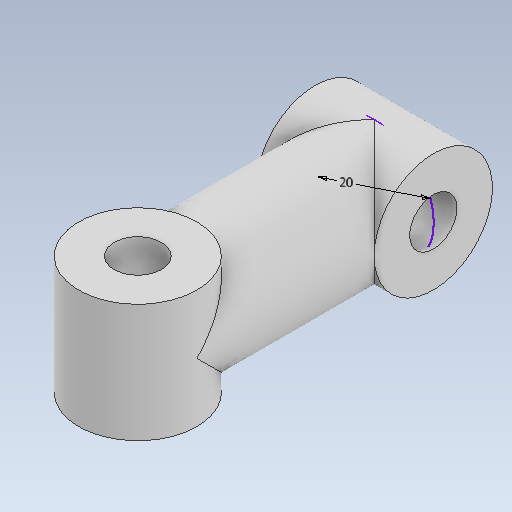
# Autodesk Inventor part: 10-06-007
Saved by Autodesk Inventor 2020 (Build 240168000, 168)
## iProperties
Created: 2019-11-09
Part Number: 10-06-007
Material: Generic
Document SubType Name: Modeling
Designer: iuliu
Density: 1 g/cm^3
Appearance: Default
Description: Suport display
Mass: 17.7888 g
Surface Area: 54.8743 cm^2
Volume: 17.7888 cm^3
Author: iuliu
Subject: 044
Autodesk Inventor part; units mm, degrees
ref_plane "YZ Plane" through (0, 0, 0) normal (1, 0, 0) x (0, 1, 0)
ref_plane "Work Plane2" through (0, 0, 10) normal (0, 0, 1) x (1, 0, 0)
sketch "Sketch2" plane through (0, 0, 10) normal (0, 0, 1) x (1, 0, 0)
  circle A0 centre (0, 0) radius 10
  dimension "d7" = 20
  constraints: 1 centre point
  measures "d7" diameter of A0
extrude "Extrusion2" add sketch "Sketch2" along normal blind 40
ref_plane "Work Plane1" through (0, -10, 0) normal (0, 1, 0) x (-1, 0, 0)
sketch "Sketch4" plane through (0, -10, 0) normal (0, 1, 0) x (-1, 0, 0)
  circle A0 centre (0, 50) radius 10
  line L0 (0, 10) -> (0, 50) projected
  line L1 (0, 10) -> (0, 50) projected
  circle A1 centre (0, 10) radius 10
  point P0 (0, 0)
  dimension "d12" = 20
  constraints: 2 centre point, 2 coincident, 1 equal radius
  measures "d12" diameter of A0
extrude "Extrusion3" add sketch "Sketch4" along normal blind 20 contours A0
sketch "Sketch5" plane through (0, 10, 50) normal (0, 1, 0) x (1, 0, 0)
  circle A0 centre (0, 0) radius 4
  point P0 (0, 50)
  dimension "d15" = 8
  constraints: 1 centre point
  measures "d15" diameter of A0
extrude "Extrusion4" cut sketch "Sketch5" against normal through all
sketch "Sketch9" plane through (0, 0, 0) normal (1, 0, 0) x (0, 1, 0)
  circle A0 centre (0, 10) radius 10
  line L0 (0, 50) -> (-10, 40) projected
  line L1 (-10, 40) -> (0, 50) projected
  line L2 (0, 50) -> (10, 40) projected
  line L3 (10, 40) -> (0, 50) projected
  line L4 (10, 10) -> (-10, 10) projected
  point P0 (0, 0)
  dimension "d39" = 20
  constraints: 2 coincident, 1 centre point, 1 midpoint
  measures "d39" diameter of A0
extrude "Extrusion8" add sketch "Sketch9" along normal mid plane 20
sketch "Sketch10" plane through (10, 0, 10) normal (1, 0, 0) x (0, 0, -1)
  circle A0 centre (0, 0) radius 4
  circle A1 centre (0, 0) radius 10 projected
  point P0 (10, 0)
  point P1 (-10, 0)
  dimension "d42" = 8
  constraints: 1 centre point, 1 concentric
  measures "d42" diameter of A0
extrude "Extrusion9" cut sketch "Sketch10" against normal through all contours A0
body "Solid1"
